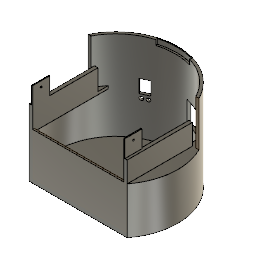
top_redesign_valueadded v6 (Autodesk Fusion 360 design; units mm, degrees)
Autodesk Fusion 360 part; units mm, degrees
sketch "Sketch1" plane through (0, 0, 0) normal (0, 0, 1) x (1, 0, 0)
  circle A0 centre (0, 0) radius 90
  line L0 (0, 0) -> (0, -55)
  line L1 (0, -55) -> (71.239, -55)
  line L2 (-71.239, -55) -> (0, -55)
  dimension "d1" = 180
  dimension "d2" = 55
  measures "d1" diameter of A0
extrude "Extrude1" add sketch "Sketch1" along normal blind 4 contours A0 L1 L2 picked at (2.1874, 41.4666)
sketch "Sketch2" plane through (0, 0, 4) normal (0, 0, 1) x (-1, 0, 0)
  line L0 (71.239, 55) -> (-71.239, 55)
  arc A0 (-71.239, 55) -> (71.239, 55) centre (0, 0) ccw
  circle A1 centre (0, 0) radius 86
extrude "Extrude2" add sketch "Sketch2" along normal blind 64 contours L0 A0 A1
sketch "Sketch3" plane through (0, 0, 4) normal (0, 0, 1) x (-1, 0, 0)
  arc A0 (-66.1135, 55) -> (66.1135, 55) centre (0, 0) ccw
  line L0 (66.1135, 55) -> (-66.1135, 55)
  line L1 (-66.1135, 55) -> (-66.1135, -55)
  arc A1 through (-66.1135, 55, 64) (0, -86, 64) (66.1135, 55, 64)
  line L2 (-66.1135, -55, 0) -> (-66.1135, -55, 64)
  arc A2 through (-66.232, 54.8573, 64) (-85.9997, -0.0928, 64.0001) (-66.1135, -55, 64.0001)
  line L3 (-66.1135, -55, 64) -> (-66.232, 54.8573, 64)
extrude "Extrude3" add sketch "Sketch3" against normal blind 4 contours A1 A2 L3 in plane through (0, 0, 68) normal (0, 0, 1)
sketch "Sketch4" plane through (0, 0, 4) normal (0, 0, 1) x (-1, 0, 0)
  arc A0 (-66.1135, 55) -> (66.1135, 55) centre (0, 0) ccw
  line L0 (66.1135, 55) -> (-66.1135, 55)
  line L1 (66.1135, 55) -> (66.1135, -55)
  arc A1 through (-66.1135, -55, 64) (55, -66.1135, 64) (66.1135, 55, 64)
  line L2 (66.1135, -55, 0) -> (66.1135, -55, 64)
  arc A2 through (66.1135, -55, 64) (86, 0, 64) (66.1135, 55, 64)
  line L3 (66.1135, -55, 64) -> (66.1135, 55, 64)
extrude "Extrude4" add sketch "Sketch4" against normal blind 4 contours A1 A2 L3 in plane through (0, 0, 68) normal (0, 0, 1)
sketch "Sketch5" plane through (0, 0, 4) normal (0, 0, 1) x (-1, 0, 0)
  arc A0 (-66.1135, 55) -> (66.1135, 55) centre (0, 0) ccw
  line L0 (66.1135, 55) -> (-66.1135, 55)
  line L1 (-71.239, 55, 64) -> (-71.239, -35, 64)
  line L2 (-66.1135, -55, 64) -> (-66.232, 54.8573, 64)
  line L3 (-71.239, -35, 64) -> (-66.1351, -35, 64)
  line L4 (71.239, 55, 64) -> (71.239, -35, 64)
  line L5 (66.1135, -55, 64) -> (66.1135, 55, 64)
  line L6 (71.239, -35, 64) -> (66.1135, -35, 64)
  line L7 (71.239, 55, 64) -> (66.1135, 55, 64)
  dimension "d12" = 90
  dimension "d13" = 90
extrude "Extrude5" add sketch "Sketch5" along normal blind 30 contours L4 L5 L6 L7 in plane through (0, 0, 68) normal (0, 0, 1)
sketch "Sketch6" plane through (0, 0, 68) normal (0, 0, 1) x (-1, 0, 0)
  line L0 (71.239, 55) -> (71.239, -35)
  line L1 (71.239, -35) -> (66.1135, -35)
  line L2 (66.1135, -35) -> (66.1135, -55)
  arc A0 (-66.1135, -55) -> (66.1135, -55) centre (0, 0) ccw
  line L3 (-66.1135, -55) -> (-66.232, 54.8573)
  arc A1 (-66.1135, 55) -> (-66.232, 54.8573) centre (0, 0) ccw
  line L4 (-66.1135, 55) -> (-71.239, 55)
  arc A2 (-71.239, 55) -> (71.239, 55) centre (0, 0) ccw
  line L5 (-71.239, 55) -> (-66.1351, 55)
  line L6 (-66.1351, 55) -> (-66.1351, -35)
  line L7 (-66.1351, -35) -> (-71.239, -35)
  line L8 (-71.239, -35) -> (-71.239, 55)
  dimension "d16" = 90
extrude "Extrude6" add sketch "Sketch6" along normal blind 30 contours L3 A1 L4 L5 L6 L7 L8
sketch "Sketch7" plane through (0, 0, 98) normal (0, 0, 1) x (-1, 0, 0)
  line L0 (-66.1351, -35) -> (-66.232, 54.8573)
  arc A0 (-66.1351, 54.9741) -> (-66.232, 54.8573) centre (0, 0) ccw
  line L1 (-66.1351, 54.9741) -> (-66.1351, 55)
  line L2 (-66.1351, 55) -> (-71.239, 55)
  line L3 (-71.239, 55) -> (-71.239, -35)
  line L4 (-71.239, -35) -> (-66.1351, -35)
  line L5 (-66.232, 54.8573) -> (-66.232, 55)
  line L6 (-66.232, 55) -> (-67.732, 55)
  line L7 (-67.732, 55) -> (-67.732, 30)
  line L8 (-67.732, 30) -> (-66.232, 30)
  line L9 (-66.232, 30) -> (-66.232, 55)
  line L10 (66.1135, 55) -> (67.6135, 55)
  line L11 (67.6135, 55) -> (67.6135, 30)
  line L12 (67.6135, 30) -> (66.1135, 30)
  line L13 (66.1135, 30) -> (66.1135, 55)
  dimension "d19" = 1.5
  dimension "d20" = 25
  dimension "d21" = 25
  dimension "d22" = 1.5
extrude "Extrude7" add sketch "Sketch7" along normal blind 25 contours L10 L11 L12 L13
sketch "Sketch8" plane through (0, 0, 98) normal (0, 0, 1) x (-1, 0, 0)
  line L0 (-66.1351, -35) -> (-66.232, 54.8573)
  arc A0 (-66.1351, 54.9741) -> (-66.232, 54.8573) centre (0, 0) ccw
  line L1 (-66.1351, 54.9741) -> (-66.1351, 55)
  line L2 (-66.1351, 55) -> (-71.239, 55)
  line L3 (-71.239, 55) -> (-71.239, -35)
  line L4 (-71.239, -35) -> (-66.1351, -35)
  line L5 (-66.232, 54.8573) -> (-66.232, 55)
  line L6 (-66.232, 55) -> (-67.732, 55)
  line L7 (-67.732, 55) -> (-67.732, 30)
  line L8 (-67.732, 30) -> (-66.232, 30)
  line L9 (-66.232, 30) -> (-66.232, 55)
  dimension "d25" = 1.5
  dimension "d26" = 25
extrude "Extrude8" add sketch "Sketch8" along normal blind 25 contours L2 L5 L6 L7 L8 L9
sketch "Sketch9" plane through (0, 0, 68) normal (0, 0, 1) x (-1, 0, 0)
  line L0 (-71.239, -35) -> (-71.239, 55)
  arc A0 (-71.239, 55) -> (71.239, 55) centre (0, 0) ccw
  line L1 (71.239, 55) -> (71.239, -35)
  line L2 (71.239, -35) -> (66.1135, -35)
  line L3 (66.1135, -35) -> (66.1135, -55)
  arc A1 (-66.1135, -55) -> (66.1135, -55) centre (0, 0) ccw
  line L4 (-66.1135, -55) -> (-66.1351, -35)
  line L5 (-66.1351, -35) -> (-71.239, -35)
  arc A2 (-66.232, 54.8573) -> (-66.1135, -55) centre (0, 0) ccw
  line L6 (-71.239, -35) -> (-78.5557, -35)
  line L7 (-78.5557, -35) -> (-82.9156, -35)
  arc A3 (66.1135, -55) -> (66.1135, 55) centre (0, 0) ccw
  line L8 (71.239, -35) -> (78.5557, -35)
  line L9 (78.5557, -35) -> (82.9156, -35)
extrude "Extrude9" add sketch "Sketch9" along normal blind 65 contours A0 A1 A2 L7 A3 L9
sketch "Sketch10" plane through (0, 0, 0) normal (0, 1, 0) x (1, 0, 0)
sketch "Sketch11" plane through (0, 0, 133) normal (0, 0, 1) x (-1, 0, 0)
  line L0 (-78.5557, -35) -> (-82.9156, -35)
  arc A0 (-82.9156, -35) -> (82.9156, -35) centre (0, 0) ccw
  line L1 (82.9156, -35) -> (78.5557, -35)
  arc A1 (-78.5557, -35) -> (78.5557, -35) centre (0, 0) ccw
  arc A2 (-24.9915, -84.898) -> (25.0041, -84.8943) centre (0, 0) ccw
  line L2 (25.0041, -84.8943) -> (0, 0)
  line L3 (0, 0) -> (-24.9915, -84.898)
  dimension "d31" = 88.5
  measures "d31" radius of A2
extrude "Extrude10" cut sketch "Sketch11" against normal blind 7.25 contours A1 A2 L2 L3
sketch "Sketch12" plane through (0, 0, 4) normal (0, 0, 1) x (-1, 0, 0)
  arc A0 (-66.1135, 55) -> (66.1135, 55) centre (0, 0) ccw
  line L0 (66.1135, 55) -> (-66.1135, 55)
  line L1 (0, 52.5) -> (68.1157, 52.5)
  line L2 (-68.1157, 52.5) -> (0, 52.5)
extrude "Extrude11" add sketch "Sketch12" along normal blind 60 contours A0 L0 L1 L2
extrude "Extrude12" add 1 faces at (22.0765, -53.3333, 64) along direction (0, 0, 1) blind 4
sketch "Sketch13" plane through (0, 0, 0) normal (1, 0, 0) x (0, 1, 0)
hole "Hole1" at (67.732, -42.503, 115.121) direction (-1, 0, 0) diameter 2.5 end through all
ref_plane "WorkPlane1" through (-45, 77.9423, 96.2822) normal (-0.5, 0.866025, 0) x (0.866025, 0.5, 0)
sketch "Sketch14" plane through (-45, 77.9423, 96.2822) normal (-0.5, 0.866025, 0) x (0.866025, 0.5, 0)
  line L0 (14.3422, 28.2822) -> (1.5422, 28.2822)
  line L1 (1.5422, 28.2822) -> (1.5422, 47.2822)
  line L2 (1.5422, 47.2822) -> (14.3422, 47.2822)
  line L3 (14.3422, 47.2822) -> (14.3422, 28.2822)
  line L4 (-84.756, 28.2822) -> (29.7747, 28.2822)
  dimension "d44" = 12.8
  dimension "d45" = 19
extrude "Extrude13" cut sketch "Sketch14" against normal blind 10
ref_plane "WorkPlane2" through (45, 77.9423, 52.8534) normal (0.5, 0.866025, 0) x (0.866025, -0.5, 0)
sketch "Sketch15" plane through (45, 77.9423, 52.8534) normal (0.5, 0.866025, 0) x (0.866025, -0.5, 0)
  line L0 (0.0337, -15.1466) -> (-24.9663, -15.1466)
  line L1 (-24.9663, -15.1466) -> (-24.9663, 14.8534)
  line L2 (-24.9663, 14.8534) -> (0.0337, 14.8534)
  line L3 (0.0337, 14.8534) -> (0.0337, -15.1466)
  line L4 (-29.756, -15.1466) -> (84.7747, -15.1466)
  dimension "d49" = 25
  dimension "d50" = 30
extrude "Extrude14" cut sketch "Sketch15" against normal blind 10
sketch "Sketch16" plane through (0, -52.5, 0) normal (0, 1, 0) x (-1, 0, 0)
  line L0 (-68.1157, 4) -> (68.1157, 4)
  line L1 (68.1157, 4) -> (68.1157, 64)
  line L2 (68.1157, 64) -> (66.1135, 64)
  line L3 (66.1135, 64) -> (66.1135, 68)
  line L4 (66.1135, 68) -> (-66.2295, 68)
  line L5 (-66.2295, 68) -> (-66.2295, 64)
  line L6 (-66.2295, 64) -> (-68.1157, 64)
  line L7 (-68.1157, 64) -> (-68.1157, 4)
ref_plane "WorkPlane7" through (-45, 77.9423, 41.3627) normal (-0.5, 0.866025, 0) x (0.866025, 0.5, 0)
move_face "OffsetFaces2" offset 11 1 faces at (22.9308, 84.1844, 38)
ref_plane "WorkPlane3" through (45, 77.9423, 40.5872) normal (0.5, 0.866025, 0) x (0.866025, -0.5, 0)
sketch "Sketch17" plane through (45, 77.9423, 40.5872) normal (0.5, 0.866025, 0) x (0.866025, -0.5, 0)
  line L0 (-24.9663, -27.4128) -> (0.0337, -27.4128)
  line L1 (0.0337, -27.4128) -> (-12.4663, -27.4128)
  line L2 (-6.2163, -27.4128) -> (-6.2163, -32.4128)
  line L3 (-24.9663, -27.4128) -> (-12.4663, -27.4128)
  line L4 (-18.7163, -27.4128) -> (-18.7163, -32.4128)
  circle A0 centre (-6.2163, -32.4128) radius 2.5
  circle A1 centre (-18.7163, -32.4128) radius 2.5
  dimension "d54" = 5
  dimension "d55" = 5
  dimension "d56" = 5
  dimension "d57" = 5
  measures "d56" diameter of A0
  measures "d57" diameter of A1
extrude "Extrude15" cut sketch "Sketch17" against normal blind 10 contours A0
ref_plane "WorkPlane4" through (45, 77.9423, 79.3393) normal (0.5, 0.866025, 0) x (0.866025, -0.5, 0)
sketch "Sketch18" plane through (45, 77.9423, 79.3393) normal (0.5, 0.866025, 0) x (0.866025, -0.5, 0)
  line L0 (-24.9663, 11.3393) -> (0.0337, 11.3393)
  line L1 (-24.9663, 11.3393) -> (-12.4663, 11.3393)
  line L2 (-18.7163, 11.3393) -> (-18.7163, 6.3393)
  circle A0 centre (-18.7163, 6.3393) radius 2.5
  dimension "d61" = 5
  dimension "d62" = 5
  measures "d62" diameter of A0
extrude "Extrude16" cut sketch "Sketch18" against normal blind 10
ref_plane "WorkPlane5" through (-80.7357, 35, 100.5) normal (0, -1, 0) x (1, 0, 0)
sketch "Sketch19" plane through (-80.7357, 35, 100.5) normal (0, -1, 0) x (1, 0, 0)
  line L0 (-5.1195, 32.5) -> (8.401, 32.5)
  line L1 (8.401, 32.5) -> (8.401, -32.5)
  line L2 (8.401, -32.5) -> (-5.1195, -32.5)
  line L3 (-5.1195, -32.5) -> (-5.1195, 32.5)
  line L4 (14.6221, -32.5) -> (2.18, -32.5)
extrude "Extrude17" cut sketch "Sketch19" against normal blind 5
extrude "Extrude18" add 1 faces at (-69.5305, 35, 78) along direction (0, 1, 0) blind 5
ref_plane "WorkPlane6" through (80.7357, 35, 100.5) normal (0, -1, 0) x (1, 0, 0)
sketch "Sketch20" plane through (80.7357, 35, 100.5) normal (0, -1, 0) x (1, 0, 0)
  line L0 (7, 33) -> (-9.4966, 33)
  line L1 (-9.4966, 33) -> (-9.4966, -32.5)
  line L2 (-9.4966, -32.5) -> (7, -32.5)
  line L3 (7, -32.5) -> (7, 33)
extrude "Extrude19" cut sketch "Sketch20" against normal blind 5
move_face "OffsetFaces1" offset 5 1 faces at (67.8364, 35, 78)
delete_face "DeleteFace1" 1 faces at (38.2213, 78.5253, 75.4994)
delete_face "DeleteFace2" 1 faces at (26.2151, 83.3052, 70.5109)
move_face "OffsetFaces3" offset -11 1 faces at (22.9308, 84.1844, 68)
sketch "Sketch21" plane through (-45, 77.9423, 41.3627) normal (-0.5, 0.866025, 0) x (0.866025, 0.5, 0)
ref_plane "WorkPlane8" through (-45, 77.9423, 90.4861) normal (-0.5, 0.866025, 0) x (0.866025, 0.5, 0)
sketch "Sketch22" plane through (-45, 77.9423, 90.4861) normal (-0.5, 0.866025, 0) x (0.866025, 0.5, 0)
  line L0 (1.5422, 22.4861) -> (14.3422, 22.4861)
  line L1 (14.3422, 22.4861) -> (11.8422, 22.4861)
  line L2 (11.8422, 22.4861) -> (11.8422, 16.9861)
  circle A0 centre (11.8422, 16.9861) radius 2.5
  dimension "d78" = 2.5
  dimension "d79" = 5.5
  dimension "d80" = 5
  measures "d80" diameter of A0
extrude "Extrude20" cut sketch "Sketch22" against normal blind 10
ref_plane "WorkPlane9" through (-45, 77.9423, 73.7883) normal (-0.5, 0.866025, 0) x (0.866025, 0.5, 0)
sketch "Sketch23" plane through (-45, 77.9423, 73.7883) normal (-0.5, 0.866025, 0) x (0.866025, 0.5, 0)
  line L0 (-84.756, 5.7883) -> (29.7747, 5.7883)
  line L1 (1.5422, 5.7883) -> (4.0422, 5.7883)
  line L2 (4.0422, 5.7883) -> (4.0422, 0.2883)
  circle A0 centre (4.0422, 0.2883) radius 2.5
  dimension "d84" = 2.5
  dimension "d85" = 5.5
  dimension "d86" = 5
  measures "d86" diameter of A0
extrude "Extrude21" cut sketch "Sketch23" against normal blind 10
sketch "Sketch24" plane through (0, 40, 0) normal (0, -1, 0) x (1, 0, 0)
  line L0 (80.6226, 68) -> (80.6226, 133)
  line L1 (80.6226, 133) -> (76.1315, 133)
  line L2 (76.1315, 133) -> (76.1315, 68)
  line L3 (76.1315, 68) -> (80.6226, 68)
ref_plane "WorkPlane10" through (0, -55, 61.5) normal (0, -1, 0) x (1, 0, 0)
sketch "Sketch25" plane through (0, -55, 61.5) normal (0, -1, 0) x (1, 0, 0)
move_face "OffsetFaces4" offset -0.097 1 faces at (66.1351, -54.9914, 88)
delete_face "DeleteFace3" 1 faces at (-33.1169, 80.8104, 71.0027)
delete_face "DeleteFace4" 1 faces at (-39.5867, 77.846, 75.9275)
move_face "OffsetFaces5" offset -11 1 faces at (-31.9799, 81.2451, 68)
move_face "OffsetFaces6" offset 11 1 faces at (-31.9799, 81.2451, 49)
ref_plane "WorkPlane11" through (-45, 77.9423, 124.0533) normal (-0.5, 0.866025, 0) x (0.866025, 0.5, 0)
sketch "Sketch26" plane through (-45, 77.9423, 124.0533) normal (-0.5, 0.866025, 0) x (0.866025, 0.5, 0)
  line L0 (1.5422, 64.0533) -> (14.3422, 64.0533)
  line L1 (14.3422, 64.0533) -> (11.8422, 64.0533)
  line L2 (11.8422, 64.0533) -> (11.8422, 69.5533)
  circle A0 centre (11.8422, 69.5533) radius 2.5
  dimension "d94" = 2.5
  dimension "d95" = 5.5
  dimension "d96" = 5
  measures "d96" diameter of A0
extrude "Extrude22" cut sketch "Sketch26" against normal blind 10
ref_plane "WorkPlane12" through (-45, 77.9423, 52.3587) normal (-0.5, 0.866025, 0) x (0.866025, 0.5, 0)
sketch "Sketch27" plane through (-45, 77.9423, 52.3587) normal (-0.5, 0.866025, 0) x (0.866025, 0.5, 0)
  line L0 (1.5422, -7.6413) -> (14.3422, -7.6413)
  line L1 (1.5422, -7.6413) -> (4.0422, -7.6413)
  line L2 (4.0422, -7.6413) -> (4.0422, -2.1413)
  circle A0 centre (4.0422, -2.1413) radius 2.5
  dimension "d100" = 2.5
  dimension "d101" = 5.5
  dimension "d102" = 5
  measures "d102" diameter of A0
extrude "Extrude23" cut sketch "Sketch27" against normal blind 10
